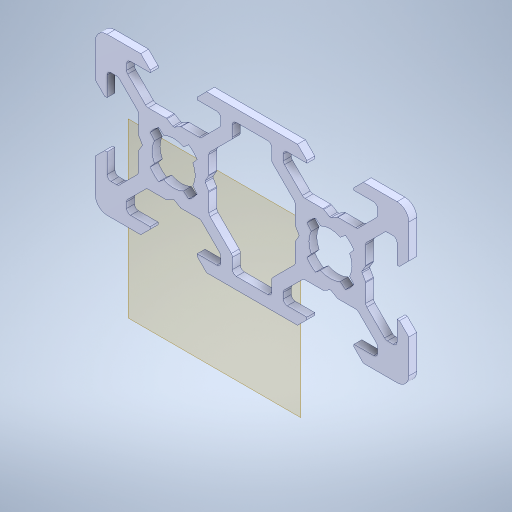
# Autodesk Inventor part: 2040Vslot
Saved by Autodesk Inventor 2023 (Build 270158000, 158)
## iProperties
Created: 2022-03-13
Part Number: 2040Vslot
Material: Generic
Description: STEP AP214
Document SubType Name: Modeling
Designer: Felix
Density: 1 g/cm^3
Appearance: Default
Sending System: SolidWorks 2018
Preprocessor: SwSTEP 2.0
Title: 2040x100 Vslot.STEP
Revision Number: ANY
Autodesk Inventor part; units mm, degrees
ref_plane "YZ Plane" through (0, 0, 0) normal (1, 0, 0) x (0, 1, 0)
ref_plane "XZ Plane" through (0, 0, 0) normal (0, 1, 0) x (-1, 0, 0)
ref_plane "XY Plane" through (0, 0, 0) normal (0, 0, 1) x (1, 0, 0)
ref_plane "Work Plane3" through (0.5, 0, 50) normal (0, 0, 1) x (1, 0, 0)
sketch "Sketch1" plane through (0.5, 0, 50) normal (0, 0, 1) x (1, 0, 0)
  arc A0 (-12.7, 20) -> (-14.2, 18.5) centre (-12.7, 18.5) ccw projected
  line L0 (-14.2, 18.5) -> (-14.2, 14.2) projected
  line L1 (-14.2, 14.2) -> (-13, 13) projected
  line L2 (-13, 13) -> (-12.7, 13) projected
  line L3 (-12.7, 13) -> (-12.7, 15.5) projected
  arc A1 (-12.2, 16) -> (-12.7, 15.5) centre (-12.2, 15.5) ccw projected
  line L4 (-12.2, 16) -> (-11.4678, 16) projected
  arc A2 (-11.1142, 15.8536) -> (-11.4678, 16) centre (-11.4678, 15.5) ccw projected
  line L5 (-11.1142, 15.8536) -> (-8.8464, 13.5858) projected
  arc A3 (-8.7, 13.2322) -> (-8.8464, 13.5858) centre (-9.2, 13.2322) ccw projected
  line L6 (-8.7, 13.2322) -> (-8.7, 10.9536) projected
  arc A4 (-8.7, 10.9536) -> (-8.6732, 10.8536) centre (-8.5, 10.9536) ccw projected
  line L7 (-8.6732, 10.8536) -> (-8.2381, 10.1) projected
  arc A5 (-8.2381, 9.9) -> (-8.2381, 10.1) centre (-8.4113, 10) ccw projected
  line L8 (-8.2381, 9.9) -> (-8.6732, 9.1464) projected
  arc A6 (-8.6732, 9.1464) -> (-8.7, 9.0464) centre (-8.5, 9.0464) ccw projected
  line L9 (-8.7, 9.0464) -> (-8.7, 6.7678) projected
  arc A7 (-8.8464, 6.4142) -> (-8.7, 6.7678) centre (-9.2, 6.7678) ccw projected
  line L10 (-8.8464, 6.4142) -> (-11.1142, 4.1464) projected
  arc A8 (-11.4678, 4) -> (-11.1142, 4.1464) centre (-11.4678, 4.5) ccw projected
  line L11 (-11.4678, 4) -> (-12.2, 4) projected
  arc A9 (-12.7, 4.5) -> (-12.2, 4) centre (-12.2, 4.5) ccw projected
  line L12 (-12.7, 4.5) -> (-12.7, 7) projected
  line L13 (-12.7, 7) -> (-13, 7) projected
  line L14 (-13, 7) -> (-14.2, 5.8) projected
  line L15 (-14.2, 5.8) -> (-14.2, 1.5) projected
  arc A10 (-14.2, 1.5) -> (-12.7, 0) centre (-12.7, 1.5) ccw projected
  line L16 (-12.7, 0) -> (-8.4, 0) projected
  line L17 (-8.4, 0) -> (-7.2, 1.2) projected
  line L18 (-7.2, 1.2) -> (-7.2, 1.5) projected
  line L19 (-7.2, 1.5) -> (-9.7, 1.5) projected
  arc A11 (-10.2, 2) -> (-9.7, 1.5) centre (-9.7, 2) ccw projected
  line L20 (-10.2, 2) -> (-10.2, 2.7322) projected
  arc A12 (-10.0536, 3.0858) -> (-10.2, 2.7322) centre (-9.7, 2.7322) ccw projected
  line L21 (-10.0536, 3.0858) -> (-7.7858, 5.3536) projected
  arc A13 (-7.4322, 5.5) -> (-7.7858, 5.3536) centre (-7.4322, 5) ccw projected
  line L22 (-7.4322, 5.5) -> (-5.1536, 5.5) projected
  arc A14 (-5.1536, 5.5) -> (-5.0536, 5.5268) centre (-5.1536, 5.7) ccw projected
  line L23 (-5.0536, 5.5268) -> (-4.3, 5.9619) projected
  arc A15 (-4.1, 5.9619) -> (-4.3, 5.9619) centre (-4.2, 5.7887) ccw projected
  line L24 (-4.1, 5.9619) -> (-3.3464, 5.5268) projected
  arc A16 (-3.3464, 5.5268) -> (-3.2464, 5.5) centre (-3.2464, 5.7) ccw projected
  line L25 (-3.2464, 5.5) -> (-0.9678, 5.5) projected
  arc A17 (-0.6142, 5.3536) -> (-0.9678, 5.5) centre (-0.9678, 5) ccw projected
  line L26 (-0.6142, 5.3536) -> (1.6536, 3.0858) projected
  arc A18 (1.8, 2.7322) -> (1.6536, 3.0858) centre (1.3, 2.7322) ccw projected
  line L27 (1.8, 2.7322) -> (1.8, 2) projected
  arc A19 (1.3, 1.5) -> (1.8, 2) centre (1.3, 2) ccw projected
  line L28 (1.3, 1.5) -> (-1.2, 1.5) projected
  line L29 (-1.2, 1.5) -> (-1.2, 1.2) projected
  line L30 (-1.2, 1.2) -> (0, 0) projected
  line L31 (0, 0) -> (11.6, 0) projected
  line L32 (11.6, 0) -> (12.8, 1.2) projected
  line L33 (12.8, 1.2) -> (12.8, 1.5) projected
  line L34 (12.8, 1.5) -> (10.3, 1.5) projected
  arc A20 (9.8, 2) -> (10.3, 1.5) centre (10.3, 2) ccw projected
  line L35 (9.8, 2) -> (9.8, 2.7322) projected
  arc A21 (9.9464, 3.0858) -> (9.8, 2.7322) centre (10.3, 2.7322) ccw projected
  line L36 (9.9464, 3.0858) -> (12.2142, 5.3536) projected
  arc A22 (12.5678, 5.5) -> (12.2142, 5.3536) centre (12.5678, 5) ccw projected
  line L37 (12.5678, 5.5) -> (14.8464, 5.5) projected
  arc A23 (14.8464, 5.5) -> (14.9464, 5.5268) centre (14.8464, 5.7) ccw projected
  line L38 (14.9464, 5.5268) -> (15.7, 5.9619) projected
  arc A24 (15.9, 5.9619) -> (15.7, 5.9619) centre (15.8, 5.7887) ccw projected
  line L39 (15.9, 5.9619) -> (16.6536, 5.5268) projected
  arc A25 (16.6536, 5.5268) -> (16.7536, 5.5) centre (16.7536, 5.7) ccw projected
  line L40 (16.7536, 5.5) -> (19.0322, 5.5) projected
  arc A26 (19.3858, 5.3536) -> (19.0322, 5.5) centre (19.0322, 5) ccw projected
  line L41 (19.3858, 5.3536) -> (21.6536, 3.0858) projected
  arc A27 (21.8, 2.7322) -> (21.6536, 3.0858) centre (21.3, 2.7322) ccw projected
  line L42 (21.8, 2.7322) -> (21.8, 2) projected
  arc A28 (21.3, 1.5) -> (21.8, 2) centre (21.3, 2) ccw projected
  line L43 (21.3, 1.5) -> (18.8, 1.5) projected
  line L44 (18.8, 1.5) -> (18.8, 1.2) projected
  line L45 (18.8, 1.2) -> (20, 0) projected
  line L46 (20, 0) -> (24.3, 0) projected
  arc A29 (24.3, 0) -> (25.8, 1.5) centre (24.3, 1.5) ccw projected
  line L47 (25.8, 1.5) -> (25.8, 5.8) projected
  line L48 (25.8, 5.8) -> (24.6, 7) projected
  line L49 (24.6, 7) -> (24.3, 7) projected
  line L50 (24.3, 7) -> (24.3, 4.5) projected
  arc A30 (23.8, 4) -> (24.3, 4.5) centre (23.8, 4.5) ccw projected
  line L51 (23.8, 4) -> (23.0678, 4) projected
  arc A31 (22.7142, 4.1464) -> (23.0678, 4) centre (23.0678, 4.5) ccw projected
  line L52 (22.7142, 4.1464) -> (20.4464, 6.4142) projected
  arc A32 (20.3, 6.7678) -> (20.4464, 6.4142) centre (20.8, 6.7678) ccw projected
  line L53 (20.3, 6.7678) -> (20.3, 9.0464) projected
  arc A33 (20.3, 9.0464) -> (20.2732, 9.1464) centre (20.1, 9.0464) ccw projected
  line L54 (20.2732, 9.1464) -> (19.8381, 9.9) projected
  arc A34 (19.8381, 10.1) -> (19.8381, 9.9) centre (20.0113, 10) ccw projected
  line L55 (19.8381, 10.1) -> (20.2732, 10.8536) projected
  arc A35 (20.2732, 10.8536) -> (20.3, 10.9536) centre (20.1, 10.9536) ccw projected
  line L56 (20.3, 10.9536) -> (20.3, 13.2322) projected
  arc A36 (20.4464, 13.5858) -> (20.3, 13.2322) centre (20.8, 13.2322) ccw projected
  line L57 (20.4464, 13.5858) -> (22.7142, 15.8536) projected
  arc A37 (23.0678, 16) -> (22.7142, 15.8536) centre (23.0678, 15.5) ccw projected
  line L58 (23.0678, 16) -> (23.8, 16) projected
  arc A38 (24.3, 15.5) -> (23.8, 16) centre (23.8, 15.5) ccw projected
  line L59 (24.3, 15.5) -> (24.3, 13) projected
  line L60 (24.3, 13) -> (24.6, 13) projected
  line L61 (24.6, 13) -> (25.8, 14.2) projected
  line L62 (25.8, 14.2) -> (25.8, 18.5) projected
  arc A39 (25.8, 18.5) -> (24.3, 20) centre (24.3, 18.5) ccw projected
  line L63 (24.3, 20) -> (20, 20) projected
  line L64 (20, 20) -> (18.8, 18.8) projected
  line L65 (18.8, 18.8) -> (18.8, 18.5) projected
  line L66 (18.8, 18.5) -> (21.3, 18.5) projected
  arc A40 (21.8, 18) -> (21.3, 18.5) centre (21.3, 18) ccw projected
  line L67 (21.8, 18) -> (21.8, 17.2678) projected
  arc A41 (21.6536, 16.9142) -> (21.8, 17.2678) centre (21.3, 17.2678) ccw projected
  line L68 (21.6536, 16.9142) -> (19.3858, 14.6464) projected
  arc A42 (19.0322, 14.5) -> (19.3858, 14.6464) centre (19.0322, 15) ccw projected
  line L69 (19.0322, 14.5) -> (16.7536, 14.5) projected
  arc A43 (16.7536, 14.5) -> (16.6536, 14.4732) centre (16.7536, 14.3) ccw projected
  line L70 (16.6536, 14.4732) -> (15.9, 14.0381) projected
  arc A44 (15.7, 14.0381) -> (15.9, 14.0381) centre (15.8, 14.2113) ccw projected
  line L71 (15.7, 14.0381) -> (14.9464, 14.4732) projected
  arc A45 (14.9464, 14.4732) -> (14.8464, 14.5) centre (14.8464, 14.3) ccw projected
  line L72 (14.8464, 14.5) -> (12.5678, 14.5) projected
  arc A46 (12.2142, 14.6464) -> (12.5678, 14.5) centre (12.5678, 15) ccw projected
  line L73 (12.2142, 14.6464) -> (9.9464, 16.9142) projected
  arc A47 (9.8, 17.2678) -> (9.9464, 16.9142) centre (10.3, 17.2678) ccw projected
  line L74 (9.8, 17.2678) -> (9.8, 18) projected
  arc A48 (10.3, 18.5) -> (9.8, 18) centre (10.3, 18) ccw projected
  line L75 (10.3, 18.5) -> (12.8, 18.5) projected
  line L76 (12.8, 18.5) -> (12.8, 18.8) projected
  line L77 (12.8, 18.8) -> (11.6, 20) projected
  line L78 (11.6, 20) -> (0, 20) projected
  line L79 (0, 20) -> (-1.2, 18.8) projected
  line L80 (-1.2, 18.8) -> (-1.2, 18.5) projected
  line L81 (-1.2, 18.5) -> (1.3, 18.5) projected
  arc A49 (1.8, 18) -> (1.3, 18.5) centre (1.3, 18) ccw projected
  line L82 (1.8, 18) -> (1.8, 17.2678) projected
  arc A50 (1.6536, 16.9142) -> (1.8, 17.2678) centre (1.3, 17.2678) ccw projected
  line L83 (1.6536, 16.9142) -> (-0.6142, 14.6464) projected
  arc A51 (-0.9678, 14.5) -> (-0.6142, 14.6464) centre (-0.9678, 15) ccw projected
  line L84 (-0.9678, 14.5) -> (-3.2464, 14.5) projected
  arc A52 (-3.2464, 14.5) -> (-3.3464, 14.4732) centre (-3.2464, 14.3) ccw projected
  line L85 (-3.3464, 14.4732) -> (-4.1, 14.0381) projected
  arc A53 (-4.3, 14.0381) -> (-4.1, 14.0381) centre (-4.2, 14.2113) ccw projected
  line L86 (-4.3, 14.0381) -> (-5.0536, 14.4732) projected
  arc A54 (-5.0536, 14.4732) -> (-5.1536, 14.5) centre (-5.1536, 14.3) ccw projected
  line L87 (-5.1536, 14.5) -> (-7.4322, 14.5) projected
  arc A55 (-7.7858, 14.6464) -> (-7.4322, 14.5) centre (-7.4322, 15) ccw projected
  line L88 (-7.7858, 14.6464) -> (-10.0536, 16.9142) projected
  arc A56 (-10.2, 17.2678) -> (-10.0536, 16.9142) centre (-9.7, 17.2678) ccw projected
  line L89 (-10.2, 17.2678) -> (-10.2, 18) projected
  arc A57 (-9.7, 18.5) -> (-10.2, 18) centre (-9.7, 18) ccw projected
  line L90 (-9.7, 18.5) -> (-7.2, 18.5) projected
  line L91 (-7.2, 18.5) -> (-7.2, 18.8) projected
  line L92 (-7.2, 18.8) -> (-8.4, 20) projected
  line L93 (-8.4, 20) -> (-12.7, 20) projected
  line L94 (17.0582, 7.5547) -> (17.7099, 7.0078) projected
  arc A58 (14.5418, 7.5547) -> (17.0582, 7.5547) centre (15.8, 10) ccw projected
  line L95 (13.8901, 7.0078) -> (14.5418, 7.5547) projected
  arc A59 (12.8104, 8.0861) -> (13.8901, 7.0078) centre (15.8, 10) ccw projected
  line L96 (13.3547, 8.7418) -> (12.8104, 8.0861) projected
  arc A60 (13.3547, 11.2582) -> (13.3547, 8.7418) centre (15.8, 10) ccw projected
  line L97 (12.8104, 11.9139) -> (13.3547, 11.2582) projected
  arc A61 (13.8901, 12.9922) -> (12.8104, 11.9139) centre (15.8, 10) ccw projected
  line L98 (14.5418, 12.4453) -> (13.8901, 12.9922) projected
  arc A62 (17.0582, 12.4453) -> (14.5418, 12.4453) centre (15.8, 10) ccw projected
  line L99 (17.7099, 12.9922) -> (17.0582, 12.4453) projected
  arc A63 (18.7896, 11.9139) -> (17.7099, 12.9922) centre (15.8, 10) ccw projected
  line L100 (18.2453, 11.2582) -> (18.7896, 11.9139) projected
  arc A64 (18.2453, 8.7418) -> (18.2453, 11.2582) centre (15.8, 10) ccw projected
  line L101 (18.7896, 8.0861) -> (18.2453, 8.7418) projected
  arc A65 (17.7099, 7.0078) -> (18.7896, 8.0861) centre (15.8, 10) ccw projected
  line L102 (-2.9418, 7.5547) -> (-2.2901, 7.0078) projected
  arc A66 (-5.4582, 7.5547) -> (-2.9418, 7.5547) centre (-4.2, 10) ccw projected
  line L103 (-6.1099, 7.0078) -> (-5.4582, 7.5547) projected
  arc A67 (-7.1896, 8.0861) -> (-6.1099, 7.0078) centre (-4.2, 10) ccw projected
  line L104 (-6.6453, 8.7418) -> (-7.1896, 8.0861) projected
  arc A68 (-6.6453, 11.2582) -> (-6.6453, 8.7418) centre (-4.2, 10) ccw projected
  line L105 (-7.1896, 11.9139) -> (-6.6453, 11.2582) projected
  arc A69 (-6.1099, 12.9922) -> (-7.1896, 11.9139) centre (-4.2, 10) ccw projected
  line L106 (-5.4582, 12.4453) -> (-6.1099, 12.9922) projected
  arc A70 (-2.9418, 12.4453) -> (-5.4582, 12.4453) centre (-4.2, 10) ccw projected
  line L107 (-2.2901, 12.9922) -> (-2.9418, 12.4453) projected
  arc A71 (-1.2104, 11.9139) -> (-2.2901, 12.9922) centre (-4.2, 10) ccw projected
  line L108 (-1.7547, 11.2582) -> (-1.2104, 11.9139) projected
  arc A72 (-1.7547, 8.7418) -> (-1.7547, 11.2582) centre (-4.2, 10) ccw projected
  line L109 (-1.2104, 8.0861) -> (-1.7547, 8.7418) projected
  arc A73 (-2.2901, 7.0078) -> (-1.2104, 8.0861) centre (-4.2, 10) ccw projected
  line L110 (3.8, 1.5) -> (7.8, 1.5) projected
  arc A74 (3.3, 2) -> (3.8, 1.5) centre (3.8, 2) ccw projected
  line L111 (3.3, 3.3536) -> (3.3, 2) projected
  arc A75 (3.3, 3.3536) -> (3.1536, 3.7071) centre (2.8, 3.3536) ccw projected
  line L112 (0.4464, 6.4142) -> (3.1536, 3.7071) projected
  arc A76 (0.3, 6.7678) -> (0.4464, 6.4142) centre (0.8, 6.7678) ccw projected
  line L113 (0.3, 9.0464) -> (0.3, 6.7678) projected
  arc A77 (0.3, 9.0464) -> (0.2732, 9.1464) centre (0.1, 9.0464) ccw projected
  line L114 (-0.1619, 9.9) -> (0.2732, 9.1464) projected
  arc A78 (-0.1619, 10.1) -> (-0.1619, 9.9) centre (0.0113, 10) ccw projected
  line L115 (0.2732, 10.8536) -> (-0.1619, 10.1) projected
  arc A79 (0.2732, 10.8536) -> (0.3, 10.9536) centre (0.1, 10.9536) ccw projected
  line L116 (0.3, 13.2322) -> (0.3, 10.9536) projected
  arc A80 (0.4464, 13.5858) -> (0.3, 13.2322) centre (0.8, 13.2322) ccw projected
  line L117 (3.1536, 16.2929) -> (0.4464, 13.5858) projected
  arc A81 (3.1536, 16.2929) -> (3.3, 16.6464) centre (2.8, 16.6464) ccw projected
  line L118 (3.3, 18) -> (3.3, 16.6464) projected
  arc A82 (3.8, 18.5) -> (3.3, 18) centre (3.8, 18) ccw projected
  line L119 (7.8, 18.5) -> (3.8, 18.5) projected
  arc A83 (8.3, 18) -> (7.8, 18.5) centre (7.8, 18) ccw projected
  line L120 (8.3, 16.6464) -> (8.3, 18) projected
  arc A84 (8.3, 16.6464) -> (8.4464, 16.2929) centre (8.8, 16.6464) ccw projected
  line L121 (11.1536, 13.5858) -> (8.4464, 16.2929) projected
  arc A85 (11.3, 13.2322) -> (11.1536, 13.5858) centre (10.8, 13.2322) ccw projected
  line L122 (11.3, 10.9536) -> (11.3, 13.2322) projected
  arc A86 (11.3, 10.9536) -> (11.3268, 10.8536) centre (11.5, 10.9536) ccw projected
  line L123 (11.7619, 10.1) -> (11.3268, 10.8536) projected
  arc A87 (11.7619, 9.9) -> (11.7619, 10.1) centre (11.5887, 10) ccw projected
  line L124 (11.3268, 9.1464) -> (11.7619, 9.9) projected
  arc A88 (11.3268, 9.1464) -> (11.3, 9.0464) centre (11.5, 9.0464) ccw projected
  line L125 (11.3, 6.7678) -> (11.3, 9.0464) projected
  arc A89 (11.1536, 6.4142) -> (11.3, 6.7678) centre (10.8, 6.7678) ccw projected
  line L126 (8.4464, 3.7071) -> (11.1536, 6.4142) projected
  arc A90 (8.4464, 3.7071) -> (8.3, 3.3536) centre (8.8, 3.3536) ccw projected
  line L127 (8.3, 2) -> (8.3, 3.3536) projected
  arc A91 (7.8, 1.5) -> (8.3, 2) centre (7.8, 2) ccw projected
  point P0 (-0.5, 0)
extrude "Extrusion1" add sketch "Sketch1" along normal blind 1
equation "\"d0\" = LENGTH"
equation "\"LENGTH\" = 1"
body "Solid2"
